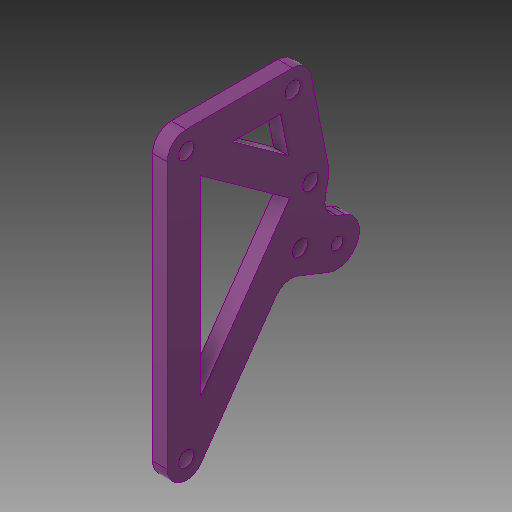
# Autodesk Inventor part: outside carriage plate
Saved by Autodesk Inventor 2017 SP1 (Build 210196100, 196)
## iProperties
Created: 2018-01-19
Part Number: outside carriage plate
Material: Aluminum 6061
Document SubType Name: Modeling
Designer: Ben
Density: 2.7 g/cm^3
Appearance: Smooth - Purple
Mass: 87.2672 g
Surface Area: 150.219 cm^2
Volume: 32.3212 cm^3
Author: Ben
Autodesk Inventor part; units mm, degrees
ref_plane "YZ Plane" through (0, 0, 0) normal (1, 0, 0) x (0, 1, 0)
ref_plane "XZ Plane" through (0, 0, 0) normal (0, 1, 0) x (-1, 0, 0)
ref_plane "XY Plane" through (0, 0, 0) normal (0, 0, 1) x (1, 0, 0)
sketch "Sketch1" plane through (0, 0, 0) normal (1, 0, 0) x (0, 1, 0)
  line L0 (-420.7503, 12.7) -> (420.7488, 12.7) construction
  line L1 (420.7488, 12.7) -> (420.7488, -12.7) construction
  line L2 (420.7488, -12.7) -> (-420.7503, -12.7) construction
  line L3 (-420.7503, -12.7) -> (-420.7503, 12.7) construction
  line L4 (0, 0) -> (0, -26.6192) construction
  circle A0 centre (0, -26.6192) radius 3.302
  circle A1 centre (38.1, 26.6192) radius 3.302
  circle A2 centre (-76.2, 26.6192) radius 3.302
  line L5 (38.1, 26.6192) -> (-76.2, 26.6192) construction
  line L6 (0, 0) -> (0, 26.6192) construction
  circle A3 centre (0, -26.6192) radius 15.875 construction
  circle A4 centre (38.1, 26.6192) radius 15.875 construction
  circle A5 centre (-76.2, 26.6192) radius 15.875 construction
  line L7 (0, -26.6192) -> (-76.2, 26.6192) construction
  arc A6 (46.1645, 26.6192) -> (38.1, 34.6837) centre (38.1, 26.6192) ccw
  arc A7 (-76.2, 34.6837) -> (-80.8188, 20.0084) centre (-76.2, 26.6192) ccw
  line L8 (-84.2645, 10.7442) -> (-84.2645, 26.6192) construction
  line L9 (-76.2, 26.6192) -> (-76.2, 0) construction
  line L10 (38.1, 26.6192) -> (38.1, 0) construction
  line L11 (45.486, 0) -> (-84.2645, 0) construction
  line L12 (-84.2645, 0) -> (-420.7503, 0) construction
  line L13 (0, -26.6192) -> (38.1, 26.6192) construction
  line L14 (0, -26.6192) -> (0, -52.0192) construction
  line L15 (13.9446, -26.6192) -> (-16.4809, -26.6192) construction
  circle A8 centre (38.1, -19.05) radius 3.302
  line L16 (38.1, -19.05) -> (38.1, 0) construction
  arc A9 (39.6714, -26.9599) -> (46.1645, -19.05) centre (38.1, -19.05) ccw
  line L17 (1.5714, -34.5291) -> (39.6714, -26.9599)
  arc A10 (-1.5642, -34.5306) -> (1.5714, -34.5291) centre (0, -26.6192) ccw
  line L18 (-76.2, 34.6837) -> (38.1, 34.6837)
  line L19 (-80.8188, 20.0084) -> (-35.1902, -11.8708)
  line L20 (0, -26.6192) -> (-22.225, -22.225) construction
  line L21 (38.1, -19.05) -> (0, -26.6192) construction
  line L22 (46.1645, 26.6192) -> (46.1645, -19.05)
  arc A11 (-32.3212, -21.4767) -> (-35.1902, -11.8708) centre (-39.8089, -18.4817) ccw
  arc A12 (-37.5367, -34.5153) -> (-19.6133, -41.6847) centre (-28.575, -38.1) ccw
  line L23 (-9.0725, -33.046) -> (-1.5642, -34.5306)
  line L24 (-32.3212, -21.4767) -> (-37.5367, -34.5153)
  line L25 (-22.225, -22.225) -> (-28.575, -38.1) construction
  line L26 (-19.6133, -41.6847) -> (-18.1244, -37.9623)
  arc A13 (-9.0725, -33.046) -> (-18.1244, -37.9623) centre (-10.6367, -40.9574) ccw
  circle A14 centre (-22.225, -22.225) radius 3.302
  circle A15 centre (-28.575, -38.1) radius 2.54
  circle A16 centre (-28.575, -38.1) radius 3.302 construction
  point P0 (0, -42.4942)
  dimension "d3" = 31.75
  dimension "d0" = 25.4
  dimension "d1" = 6.604
  dimension "d2" = 13.9192
  dimension "d4" = 38.1
  dimension "d5" = 76.2
  dimension "d10" = 25.4
  dimension "d14" = 6.35
  dimension "d59" = 4.7625
  dimension "d62" = 22.225
  dimension "d63" = 22.225
  dimension "d65" = 28.575
  dimension "d66" = 38.1
  dimension "d67" = 5.08
  dimension "d68" = 6.35
  constraints: 54 end point, 16 centre point, 15 coincident, 15 point on circle, 12 tangent, 10 equal radius, 8 parallel, 7 point on line, 7 vertical, 3 horizontal, 3 perpendicular, 2 collinear, 1 midpoint, 1 vertical alignment, 4 other
  measures "d0" distance of L0.end L1.end
  measures "d1" diameter of A0
  measures "d2" distance from line of L2 L4.end
  measures "d4" horizontal distance of L5.start L4.end
  measures "d5" distance from line of A2.centre L6
  measures "d10" distance of L13.start L14.end
  measures "d14" distance from line of L2 L16.start
  measures "d59" radial gap between concentric circles of A1 A6
  measures "d62" distance from line of L4 L20.end
  measures "d63" distance from line of L11 L20.end
  measures "d65" distance from line of L4 A12.centre
  measures "d66" distance from line of L11 A12.centre
  measures "d67" diameter of A15
  measures "d68" radial gap between concentric circles of A12 A16
extrude "Extrusion1" add sketch "Sketch1" along normal blind 6.35
sketch "Sketch5" plane through (0, 0, 0) normal (-1, 0, 0) x (0, 0, 1)
  circle A0 centre (-19.05, 38.1) radius 3.302 construction
  circle A1 centre (26.6192, -76.2) radius 3.302 construction
  circle A2 centre (26.6192, 38.1) radius 3.302 construction
  circle A3 centre (-26.6192, 0) radius 3.302 construction
  arc A4 (34.6837, 38.1) -> (26.6192, 46.1645) centre (26.6192, 38.1) ccw construction
  arc A5 (-19.05, 46.1645) -> (-26.9599, 39.6714) centre (-19.05, 38.1) ccw construction
  line L0 (-26.9599, 39.6714) -> (-34.5291, 1.5714) construction
  arc A6 (-34.5291, 1.5714) -> (-34.5306, -1.5642) centre (-26.6192, 0) ccw construction
  arc A7 (20.0084, -80.8188) -> (34.6837, -76.2) centre (26.6192, -76.2) ccw construction
  line L1 (26.6192, 38.1) -> (-26.6192, 0) construction
  circle A8 centre (26.6192, -76.2) radius 3.302 construction
  line L2 (-26.6192, 0) -> (26.6192, -76.2) construction
  circle A9 centre (26.6192, 38.1) radius 3.302 construction
  line L3 (26.6192, -76.2) -> (26.6192, 38.1) construction
  line L4 (26.6192, 38.1) -> (-19.05, 38.1) construction
  circle A10 centre (-26.6192, 0) radius 3.302 construction
  line L5 (-19.05, 38.1) -> (-26.6192, 0) construction
  line L6 (-13.8374, 31.75) -> (-17.2637, 14.5038)
  line L7 (-17.2637, 14.5038) -> (6.835, 31.75)
  line L8 (6.835, 31.75) -> (-13.8374, 31.75)
  line L9 (-3.5012, 31.75) -> (-3.5012, 38.1) construction
  line L10 (-15.5506, 23.1269) -> (-21.7788, 24.3643) construction
  line L11 (-5.2144, 23.1269) -> (-1.5188, 17.963) construction
  line L12 (20.2692, 25.7471) -> (-17.8179, -1.51)
  line L13 (-17.8179, -1.51) -> (20.2692, -56.024)
  line L14 (20.2692, -56.024) -> (20.2692, 25.7471)
  line L15 (-1.5188, 17.963) -> (2.1767, 12.7992) construction
  line L16 (20.2692, -15.1385) -> (26.6192, -15.1385) construction
  line L17 (1.2256, -28.767) -> (-3.9797, -32.4038) construction
  line L18 (26.6192, 46.1645) -> (-19.05, 46.1645) projected
  arc A11 (-11.8708, -35.1902) -> (-21.4767, -32.3212) centre (-18.4817, -39.8089) ccw projected
  line L19 (-11.8708, -35.1902) -> (20.0084, -80.8188) projected
  line L20 (34.6837, -76.2) -> (34.6837, 38.1) projected
  line L21 (-34.5306, -1.5642) -> (-33.046, -9.0725) projected
  arc A12 (-37.9623, -18.1244) -> (-33.046, -9.0725) centre (-40.9574, -10.6367) ccw projected
  line L22 (-37.9623, -18.1244) -> (-41.6847, -19.6133) projected
  arc A13 (-41.6847, -19.6133) -> (-34.5153, -37.5367) centre (-38.1, -28.575) ccw projected
  line L23 (-34.5153, -37.5367) -> (-21.4767, -32.3212) projected
  point P0 (0, 0)
  dimension "d48" = 6.35
  constraints: 34 end point, 6 midpoint, 6 perpendicular, 6 point on line, 5 equal length, 5 parallel, 2 horizontal, 2 vertical, 1 coincident
  measures "d48" distance between parallel lines of L4 L8
extrude "Extrusion2" cut sketch "Sketch5" against normal through all
body "Solid1"
